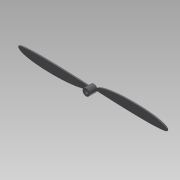
# Autodesk Inventor part: Helice 4.5x4.5
Saved by Autodesk Inventor 2016 (Build 200138000, 138)
## iProperties
Created: 2016-01-22
Part Number: Helice 4.5x4.5
Material: Plastique ABS
Document SubType Name: Modeling
Designer: sd
Mass: 0.794875 g
Surface Area: 16.8418 cm^2
Volume: 0.749882 cm^3
Density: 1.06 g/cm^3
Appearance: Lisse - Gris moyen
Author: sd
Autodesk Inventor part; units mm, degrees
ref_plane "YZ Plane" through (0, 0, 0) normal (1, 0, 0) x (0, 1, 0)
ref_plane "XZ Plane" through (0, 0, 0) normal (0, 1, 0) x (-1, 0, 0)
ref_plane "XY Plane" through (0, 0, 0) normal (0, 0, 1) x (1, 0, 0)
sketch "Esquisse1" plane through (0, 0, 0) normal (0, 1, 0) x (-1, 0, 0)
  circle A0 centre (0, 0) radius 1.25
  circle A1 centre (0, 0) radius 2.75
  dimension "d0" = 2.5
  dimension "d1" = 5.5
  constraints: 2 centre point, 2 coincident
  measures "d0" diameter of A0
  measures "d1" diameter of A1
extrude "Extrusion1" add sketch "Esquisse1" along normal blind 6
sketch "Esquisse2" plane through (0, 6, 0) normal (0, 1, 0) x (1, 0, 0)
  circle A0 centre (0, 0) radius 2.75 projected
  circle A1 centre (0, 0) radius 57.15
  spline S0 degree 3 poles (-57.15, 0) (-60.3141, 7.3699) (-9.2386, 8.3963) (-2.4495, 1.25) knots 0 0 0 0 1 1 1 1
  spline S1 degree 2 poles (-57.15, 0) (-51.1105, -2.5712) (-2.75, 0) knots 0 0 0 1 1 1
  point P0 (-55.0001, 3)
  point P1 (-25, 6)
  point P2 (-51, -1)
  dimension "d4" = 114.3
  constraints: 2 point on circle, 1 coincident, 1 horizontal alignment, 9 other
extrude "Extrusion2" add sketch "Esquisse2" against normal blind 1 contours A0 S1 A1 S0 | A1 S0 picked at (-21.1571, 1.4807)
pattern_circular "Réseau circulaire1" count 2 over 360 about axis through (0, 0, 0) along (0, -1, 0) of "Extrusion2"
